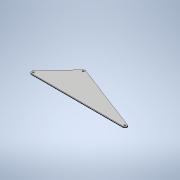
# Autodesk Inventor part: ternary link
Saved by Autodesk Inventor 2020 (Build 240168000, 168)
## iProperties
Created: 2021-02-18
Part Number: ternary link
Material: 一般
Document SubType Name: Modeling
Designer: wasd5
Density: 1 g/cm^3
Appearance: 預設
Author: wasd5
Autodesk Inventor part; units mm, degrees
ref_plane "YZ Plane" through (0, 0, 0) normal (1, 0, 0) x (0, 1, 0)
ref_plane "XZ Plane" through (0, 0, 0) normal (0, 1, 0) x (-1, 0, 0)
ref_plane "XY Plane" through (0, 0, 0) normal (0, 0, 1) x (1, 0, 0)
sketch "草圖2" plane through (0, 0, 0) normal (0, 1, 0) x (-1, 0, 0)
  line L0 (-134.8421, -144.9883) -> (0, 0) construction
  line L1 (0, 0) -> (-513, 0) construction
  arc A0 (-513, 10) -> (-516.58, -9.3372) centre (-513, 0) ccw
  arc A1 (7.3226, -6.8102) -> (0, 10) centre (0, 0) ccw
  line L2 (-513, 10) -> (0, 10)
  line L3 (-516.58, -9.3372) -> (-138.4221, -154.3255)
  line L4 (-513, 0) -> (-134.8421, -144.9883) construction
  arc A2 (-138.4221, -154.3255) -> (-127.5195, -151.7985) centre (-134.8421, -144.9883) ccw
  line L5 (7.3226, -6.8102) -> (-127.5195, -151.7985)
  circle A3 centre (-513, 0) radius 5
  circle A4 centre (0, 0) radius 5
  circle A5 centre (-134.8421, -144.9883) radius 5
  dimension "d11" = 20
  dimension "hole" = 10
  dimension "center_distance1" = 513
  dimension "center_distance3" = 405
  dimension "center_distance2" = 198
  constraints: 12 end point, 7 coincident, 6 centre point, 6 point on circle, 6 tangent, 4 equal radius, 1 horizontal
  measures "d11" diameter of A0
  measures "hole" diameter of A3
  measures "center_distance1" distance of L1.start L1.end
  measures "center_distance3" distance of L4.start L4.end
  measures "center_distance2" distance of L4.end L1.start
extrude "擠出2" add sketch "草圖2" along normal blind 5
equation "\"d11\" = 2 * hole"
